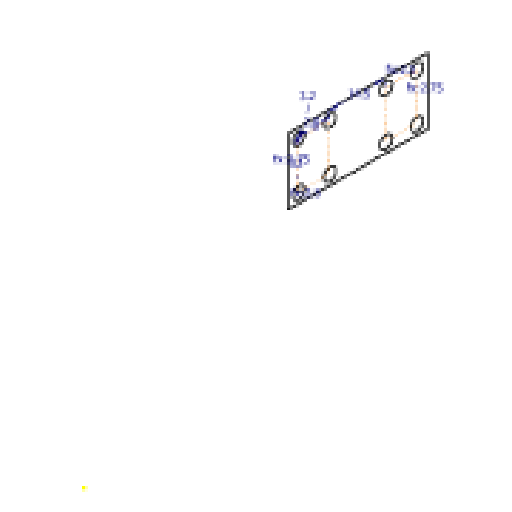
# Autodesk Inventor part: HorizontalSlidesMountingSpacer
Saved by Autodesk Inventor 2023 (Build 270158000, 158)
## iProperties
Created: 2022-11-08
Part Number: HorizontalSlidesMountingSpacer
Material: Generic
Document SubType Name: Modeling
Designer: deli
Density: 1 g/cm^3
Appearance: Default
Author: deli
Autodesk Inventor part; units mm, degrees
ref_plane "YZ Plane" through (0, 0, 0) normal (1, 0, 0) x (0, 1, 0)
ref_plane "XZ Plane" through (0, 0, 0) normal (0, 1, 0) x (-1, 0, 0)
ref_plane "XY Plane" through (0, 0, 0) normal (0, 0, 1) x (1, 0, 0)
sketch "Sketch1" plane through (0, 0, 0) normal (1, 0, 0) x (0, 1, 0)
  line L0 (53.8247, -47.1405) -> (33.8247, -47.1405)
  line L1 (33.8247, -47.1405) -> (33.8247, -94.9405)
  line L2 (33.8247, -94.9405) -> (53.8247, -94.9405)
  line L3 (53.8247, -94.9405) -> (53.8247, -47.1405)
  circle A0 centre (51.3247, -51.5905) radius 1.6
  circle A1 centre (36.3247, -51.5905) radius 1.6
  circle A2 centre (51.3247, -61.5905) radius 1.6
  circle A3 centre (36.3247, -61.5905) radius 1.6
  circle A4 centre (51.3247, -90.4905) radius 1.6
  circle A5 centre (51.3247, -80.4905) radius 1.6
  circle A6 centre (36.3247, -80.4905) radius 1.6
  circle A7 centre (36.3247, -90.4905) radius 1.6
  line L4 (51.3247, -51.5905) -> (51.3247, -61.5905) construction
  line L5 (51.3247, -61.5905) -> (36.3247, -61.5905) construction
  line L6 (36.3247, -61.5905) -> (36.3247, -51.5905) construction
  line L7 (36.3247, -51.5905) -> (51.3247, -51.5905) construction
  line L8 (51.3247, -80.4905) -> (51.3247, -90.4905) construction
  line L9 (51.3247, -90.4905) -> (36.3247, -90.4905) construction
  line L10 (36.3247, -90.4905) -> (36.3247, -80.4905) construction
  line L11 (36.3247, -80.4905) -> (51.3247, -80.4905) construction
  point P0 (0, 0)
  dimension "d0" = 3.2
  dimension "d1" = 15
  dimension "d2" = 2.5
  dimension "d3" = 2.5
  dimension "d4" = 2.5
  dimension "d5" = 10
  dimension "d6" = 4.45
  dimension "d7" = 4.45
  dimension "d8" = 18.9
  constraints: 24 end point, 9 parallel, 8 centre point, 7 equal radius, 2 equal length, 2 perpendicular, 1 coincident, 1 horizontal
  measures "d0" diameter of A0
  measures "d1" distance of L6.end L4.start
  measures "d2" distance between parallel lines of L3 L4
  measures "d3" distance between parallel lines of L1 L6
  measures "d4" distance between parallel lines of L3 L8
  measures "d5" distance of L4.start L4.end
  measures "d6" distance between parallel lines of L0 L7
  measures "d7" distance between parallel lines of L2 L9
  measures "d8" distance between parallel lines of L11 L5
extrude "Extrusion1" add sketch "Sketch1" along normal blind 3.175
equation "\"d3\" = d2"
equation "\"d4\" = d2"
equation "\"d7\" = d6"
body "Solid1"
